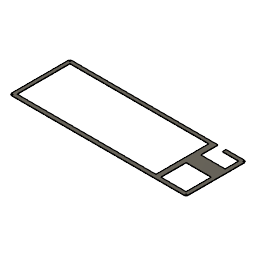
Easyboard-Case-Top (Autodesk Fusion 360 design; units mm, degrees)
part number: 2026-04-01-17-18-10-865
Autodesk Fusion 360 part; units mm, degrees
sketch "Sketch6" plane through (0, 0, 0) normal (0, 0, 1) x (1, 0, 0)
  line L0 (-20, -140) -> (430.8, -140)
  line L1 (430.8, -140) -> (430.8, -294.5)
  line L2 (430.8, -294.5) -> (-20, -294.5)
  line L3 (-20, -294.5) -> (-20, -140)
  dimension "d40" = 450.8
  dimension "d41" = 154.5
  constraint horizontal L0
  constraint vertical L1
  constraint horizontal L2
  constraint vertical L3
  measures "d40" distance of L0.start L0.end
  measures "d41" distance of L0.start L2.end
extrude "Extrude8" add sketch "Sketch6" along normal blind 1
sketch "Sketch7" plane through (0, 0, 1) normal (0, 0, 1) x (-1, 0, 0)
  line L0 (20, 294.5) -> (-430.8, 294.5)
  line L1 (-430.8, 294.5) -> (-430.8, 140)
  line L2 (-430.8, 140) -> (20, 140)
  line L3 (20, 140) -> (20, 294.5)
  line L4 (-358.09, 140) -> (-378.09, 140)
  line L5 (-378.09, 140) -> (-378.09, 184)
  line L6 (-378.09, 184) -> (-358.09, 184)
  line L7 (-358.09, 184) -> (-358.09, 140)
  line L8 (-378.09, 184) -> (-419.8, 184)
  line L9 (-419.8, 184) -> (-419.8, 149.5)
  line L10 (-419.8, 149.5) -> (-378.09, 149.5)
  line L11 (-378.09, 149.5) -> (-378.09, 184)
  line L12 (10.5, 149.5) -> (-343.5, 149.5)
  line L13 (-343.5, 149.5) -> (-343.5, 284)
  line L14 (-343.5, 284) -> (10.5, 284)
  line L15 (10.5, 284) -> (10.5, 149.5)
  line L16 (-356.3, 220) -> (-420.3, 220)
  line L17 (-420.3, 220) -> (-420.3, 284)
  line L18 (-420.3, 284) -> (-356.3, 284)
  line L19 (-356.3, 284) -> (-356.3, 220)
  circle A0 centre (-426.8, 144) radius 1.1
  circle A1 centre (-426.8, 290.5) radius 1.1
  circle A2 centre (16, 290.5) radius 1.1
  circle A3 centre (16, 144) radius 1.1
  dimension "d46" = 20
  dimension "d47" = 44
  dimension "d48" = 52.71
  dimension "d51" = 41.71
  dimension "d52" = 34.5
  dimension "d55" = 354
  dimension "d56" = 134.5
  dimension "d57" = 9.5
  dimension "d58" = 9.5
  dimension "d59" = 64
  dimension "d60" = 64
  dimension "d61" = 10.5
  dimension "d62" = 10.5
  dimension "d67" = 2.2
  dimension "d68" = 2.2
  dimension "d69" = 2.2
  dimension "d70" = 2.2
  dimension "d71" = 4
  dimension "d72" = 4
  dimension "d73" = 4
  dimension "d74" = 4
  dimension "d75" = 4
  dimension "d76" = 4
  dimension "d77" = 4
  dimension "d78" = 4
  constraint horizontal L4
  constraint vertical L5
  constraint horizontal L6
  constraint vertical L7
  constraint coincident L2 L4.start
  constraint horizontal L8
  constraint vertical L9
  constraint horizontal L10
  constraint vertical L11
  constraint horizontal L12
  constraint vertical L13
  constraint horizontal L14
  constraint vertical L15
  constraint horizontal L16
  constraint vertical L17
  constraint horizontal L18
  constraint vertical L19
  measures "d46" distance of L4.start L4.end
  measures "d47" distance of L4.start L6.end
  measures "d48" distance of L1 L5
  measures "d51" distance of L5.end L8.end
  measures "d52" distance of L5.end L10.end
  measures "d55" distance of L12.start L12.end
  measures "d56" distance of L12.start L14.end
  measures "d57" distance of L3 L15
  measures "d58" distance of L2 L12
  measures "d59" distance of L16.start L16.end
  measures "d60" distance of L16.start L18.end
  measures "d61" distance of L1 L17
  measures "d62" distance of L0 L18
  measures "d67" diameter of A0
  measures "d68" diameter of A1
  measures "d69" diameter of A2
  measures "d70" diameter of A3
  measures "d71" distance of L2 A3.centre
  measures "d72" distance of L3 A3.centre
  measures "d73" distance of L3 A2.centre
  measures "d74" distance of L0 A2.centre
  measures "d75" distance of L0 A1.centre
  measures "d76" distance of L1 A1.centre
  measures "d77" distance of L1 A0.centre
  measures "d78" distance of L2 A0.centre
extrude "Extrude9" cut sketch "Sketch7" against normal blind 1 contours L2 L4 L5 L6 L7 L11
extrude "Extrude10" cut sketch "Sketch7" against normal blind 1 contours L5 L8 L9 L10 L11
extrude "Extrude11" cut sketch "Sketch7" against normal blind 1 contours L12 L13 L14 L15 | L16 L17 L18 L19
fillet "Fillet6" radius 6 4 edges at (-20, -294.5, 0.5) (-20, -140, 0.5) (430.8, -140, 0.5) (430.8, -294.5, 0.5)
extrude "Extrude12" cut sketch "Sketch7" against normal blind 1 contours A0 | A1 | A2 | A3
equation "d51 = 52.210 mm - 10.50 mm"
equation "d52 = 44 mm - 9.5 mm"
